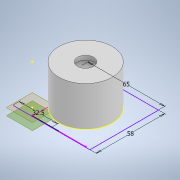
# Autodesk Inventor part: Part3
Saved by Autodesk Inventor 2020.1 (Build 241239000, 239)
## iProperties
Created: 2019-11-07
Part Number: Part3
Material: Generic
Document SubType Name: Modeling
Designer: super
Density: 1 g/cm^3
Appearance: Default
Author: super
Autodesk Inventor part; units mm, degrees
ref_plane "YZ Plane" through (0, 0, 0) normal (1, 0, 0) x (0, 1, 0)
ref_plane "XZ Plane" through (0, 0, 0) normal (0, 1, 0) x (-1, 0, 0)
ref_plane "XY Plane" through (0, 0, 0) normal (0, 0, 1) x (1, 0, 0)
ref_plane "Work Plane3" through (0, 6, 0) normal (0, 1, 0) x (1, 0, 0)
sketch "Sketch2" plane through (0, 6, 0) normal (0, 1, 0) x (1, 0, 0)
  line L0 (0, 0) -> (0, 22.5)
  line L1 (0, 45) -> (0, 0) projected
  line L2 (0, 22.5) -> (22.5, 22.5)
  circle A0 centre (22.5, 22.5) radius 22.5
  dimension "d5" = 22.5
  dimension "d6" = 22.5
  dimension "d7" = 45
  constraints: 4 end point, 1 centre point, 1 coincident, 1 midpoint, 1 perpendicular
  measures "d5" distance of L0.start L0.end
  measures "d6" distance of L0.end L2.end
  measures "d7" diameter of A0
extrude "Extrusion2" add sketch "Sketch2" along normal blind 33.5
ref_plane "Work Plane2" through (0, 0, 0) normal (0, -1, 0) x (1, 0, 0)
sketch "Sketch3" plane through (0, 0, 0) normal (0, -1, 0) x (1, 0, 0)
  line L0 (0, -45) -> (0, 0) projected
  line L1 (0, 0) -> (0, -22.5)
  circle A0 centre (22.5, -22.5) radius 18.25
  dimension "d12" = 36.5
  constraints: 2 end point, 1 centre point, 1 midpoint
  measures "d12" diameter of A0
extrude "Extrusion3" cut sketch "Sketch3" against normal blind 65
sketch "Sketch4" plane through (22.5, 39.5, -22.5) normal (0, 1, 0) x (1, 0, 0)
  circle A0 centre (0, 0) radius 6.75
  point P0 (-22.5, -22.5)
  dimension "d15" = 13.5
  constraints: 1 centre point
  measures "d15" diameter of A0
extrude "Extrusion4" cut sketch "Sketch4" against normal blind 4.5
ref_plane "Work Plane1" through (0, 0, 0) normal (0, -1, 0) x (1, 0, 0)
sketch "Sketch5" plane through (0, 0, 0) normal (0, -1, 0) x (1, 0, 0)
  line L0 (0, -45) -> (0, 0) projected
  line L1 (0, 0) -> (22.5, 0)
  line L2 (0, 0) -> (45, 0) projected
  constraints: 2 end point, 1 midpoint
sketch "Sketch6" plane through (22.5, 39.5, -22.5) normal (0, 1, 0) x (1, 0, 0)
  point P0 (-22.5, -22.5)
sketch "Sketch7" plane through (22.5, 39.5, -22.5) normal (0, 1, 0) x (1, 0, 0)
  circle A0 centre (0, 0) radius 18.25 projected
  circle A1 centre (0, 0) radius 18.25
  point P0 (-22.5, -22.5)
  constraints: 1 centre point, 1 coincident
extrude "Extrusion5" add sketch "Sketch7" against normal blind 3.5
sketch "Sketch8" plane through (22.5, 39.5, -22.5) normal (0, 1, 0) x (1, 0, 0)
  circle A0 centre (0, 0) radius 6.75
  point P0 (-22.5, -22.5)
  dimension "d20" = 13.5
  constraints: 1 centre point
  measures "d20" diameter of A0
extrude "Extrusion6" cut sketch "Sketch8" against normal blind 3.5
sketch "Sketch9" plane through (22.5, 6, -22.5) normal (0, -1, 0) x (1, 0, 0)
  point P0 (-22.5, 22.5)
sketch "Sketch10" plane through (22.5, 39.5, -22.5) normal (0, 1, 0) x (1, 0, 0)
  point P0 (-22.5, -22.5)
sketch "Sketch11" plane through (22.5, 6, -22.5) normal (0, -1, 0) x (1, 0, 0)
  circle A0 centre (0, 0) radius 22.5 projected
  line L0 (0, 29) -> (32.5, 29)
  line L1 (32.5, 29) -> (32.5, -29)
  line L2 (32.5, -29) -> (-32.5, -29)
  line L3 (0, 29) -> (-32.5, 29)
  point P0 (-22.5, 22.5)
  dimension "d25" = 58
  dimension "d26" = 65
  dimension "d27" = 32.5
  constraints: 8 end point, 2 perpendicular, 1 horizontal
  measures "d25" distance of L0.end L1.end
  measures "d26" distance of L1.end L2.end
  measures "d27" distance of L0.start L3.end
body "Solid1"
